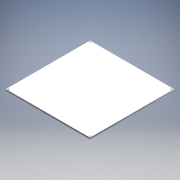
# Autodesk Inventor part: alu plate
Saved by Autodesk Inventor 2017 (Build 210142000, 142)
## iProperties
Part Number: alu plate
Material: Aluminium 6061
Document SubType Name: Modeling
Designer: Till
Density: 2.7 g/cm^3
Appearance: Aluminium - flach
Author: Till
Autodesk Inventor part; units mm, degrees
ref_plane "YZ Plane" through (0, 0, 0) normal (1, 0, 0) x (0, 1, 0)
ref_plane "XZ Plane" through (0, 0, 0) normal (0, 1, 0) x (-1, 0, 0)
ref_plane "XY Plane" through (0, 0, 0) normal (0, 0, 1) x (1, 0, 0)
sketch "Skizze1" plane through (0, 0, 0) normal (0, 0, 1) x (1, 0, 0)
  line L0 (-157.5, -157.5) -> (157.5, -157.5)
  line L1 (157.5, -157.5) -> (157.5, 157.5)
  line L2 (157.5, 157.5) -> (-157.5, 157.5)
  line L3 (-157.5, 157.5) -> (-157.5, -157.5)
  line L4 (-157.5, -157.5) -> (157.5, 157.5) construction
  line L5 (157.5, -157.5) -> (-157.5, 157.5) construction
  point P0 (0, 0)
  dimension "d0" = 315
  dimension "d1" = 315
  constraints: 12 end point, 2 midpoint, 2 parallel, 1 horizontal, 1 perpendicular
  measures "d0" distance of L2.end L1.end
  measures "d1" distance of L1.end L0.end
extrude "Extrusion1" add sketch "Skizze1" along normal blind 6
hole "Bohrung1" at (-152.5, -152.5, 6) direction (0, 0, -1) diameter 3 end through all countersink diameter 5.65 countersink angle 90
hole "Bohrung2" at (152.5, -152.5, 6) direction (0, 0, -1) diameter 3 end through all countersink diameter 5.56 countersink angle 90
hole "Bohrung3" at (152.5, 152.5, 6) direction (0, 0, -1) diameter 3 end through all countersink diameter 5.56 countersink angle 90
hole "Bohrung4" at (-152.5, 152.5, 6) direction (0, 0, -1) diameter 3 end through all countersink diameter 5.56 countersink angle 90
